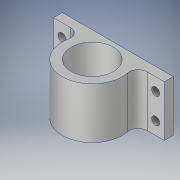
# Autodesk Inventor part: Motor Holder
Saved by Autodesk Inventor 2017 (Build 210142000, 142)
## iProperties
Created: 2017-01-31
Part Number: Motor Holder
Material: Aluminum 6061
Document SubType Name: Modeling
Designer: qupec
Density: 2.7 g/cm^3
Appearance: Aluminum - Flat
Author: qupec
Autodesk Inventor part; units mm, degrees
ref_plane "YZ Plane" through (0, 0, 0) normal (1, 0, 0) x (0, 1, 0)
ref_plane "XZ Plane" through (0, 0, 0) normal (0, 1, 0) x (-1, 0, 0)
sketch "Sketch1" plane through (0, 0, 0) normal (0, 1, 0) x (-1, 0, 0)
  circle A0 centre (0, 0) radius 7.5
  line L0 (0, -7.5) -> (0, -7.5) construction
  arc A1 (10.4644, -2.11) -> (-10.4644, -2.11) centre (0, 0) ccw
  line L1 (0, -9.0875) -> (-19.685, -9.0875)
  line L2 (-19.685, -9.0875) -> (-19.685, -5.9125)
  line L3 (-19.685, -5.9125) -> (-13.5768, -5.9125)
  arc A2 (-13.5768, -5.9125) -> (-10.4644, -2.11) centre (-13.5768, -2.7375) ccw
  line L4 (0, -9.0875) -> (0, 10.675) construction
  line L5 (0, -9.0875) -> (19.685, -9.0875)
  line L6 (19.685, -9.0875) -> (19.685, -5.9125)
  line L7 (19.685, -5.9125) -> (13.5768, -5.9125)
  arc A3 (10.4644, -2.11) -> (13.5768, -5.9125) centre (13.5768, -2.7375) ccw
  dimension "d0" = 15
  dimension "d33" = 3.175
  dimension "d34" = 1.5875
  dimension "d35" = 19.685
  dimension "d36" = 3.175
  dimension "d37" = 6.35
  constraints: 16 end point, 7 point on circle, 5 symmetric about line, 3 centre point, 2 coincident, 2 horizontal, 2 tangent, 1 perpendicular, 1 vertical, 1 vertical alignment, 3 other
  measures "d34" distance of L0.end L1.start
  measures "d35" distance of L1.start L1.end
  measures "d36" distance of L1.end L2.end
  measures "d37" diameter of A2
ref_plane "Work Plane1" through (-5.4205, 4.7625, -2.8174) normal (0, 0, 1) x (1, 0, 0)
extrude "Extrusion5" add sketch "Sketch1" along normal blind 15.5
sketch "Sketch7" plane through (0, 0, 0) normal (0, -1, 0) x (1, 0, 0)
  circle A0 centre (0, 0) radius 7.5 construction
  line L0 (-19.685, -9.0875) -> (19.685, -9.0875) projected
  line L1 (19.685, -9.0875) -> (19.685, -5.9125) projected
  line L2 (19.685, -5.9125) -> (13.5768, -5.9125) projected
  arc A1 (10.4644, -2.11) -> (13.5768, -5.9125) centre (13.5768, -2.7375) ccw projected
  arc A2 (10.4644, -2.11) -> (-10.4644, -2.11) centre (0, 0) ccw projected
  arc A3 (-13.5768, -5.9125) -> (-10.4644, -2.11) centre (-13.5768, -2.7375) ccw projected
  line L3 (-13.5768, -5.9125) -> (-19.685, -5.9125) projected
  line L4 (-19.685, -5.9125) -> (-19.685, -9.0875) projected
extrude "Extrusion6" add sketch "Sketch7" along normal blind 2.54
sketch "Sketch6" plane through (13.5768, 0, -5.9125) normal (0, 0, 1) x (1, 0, 0)
  line L0 (6.1082, 0) -> (0, 0) projected
  line L1 (6.1082, 0) -> (6.1082, 15.5) projected
  line L2 (0, 15.5) -> (0, -2.54) projected
  line L3 (-3.1124, 15.5) -> (0, 15.5) projected
  line L4 (-3.1124, 15.5) -> (-3.1124, -2.54) projected
  line L5 (0, 15.5) -> (6.1082, 15.5) projected
  line L6 (0, -2.54) -> (-3.1124, -2.54) projected
  line L7 (6.1082, -2.54) -> (0, -2.54) projected
  point P0 (-13.5768, 0)
  point P1 (3.0541, 1.97)
  point P2 (3.0541, 10.99)
  dimension "d42" = 3.0541
  dimension "d43" = 6.1082
  dimension "d44" = 3.0541
  dimension "d46" = 4.51
  dimension "d56" = 18.04
  dimension "d57" = 4.51
  measures "d42" distance from line of point (3.054, 1.97) L1
  measures "d43" distance between parallel lines of L2 L1
  measures "d44" distance from line of L1 point (3.054, 10.99)
  measures "d46" distance from line of point (3.054, 10.99) L5
  measures "d56" distance between parallel lines of L7 L5
  measures "d57" distance from line of L7 point (3.054, 1.97)
hole "Hole1" at (16.6309, 1.97, -5.9125) at (16.6309, 10.99, -5.9125) direction (0, 0, -1) diameter 2.8448 depth 25.4 tip angle 118
mirror "Mirror3" about plane through (0, 0, 0) normal (1, 0, 0) of "Hole1"
sketch "Sketch8" plane through (0, -2.54, 0) normal (0, -1, 0) x (1, 0, 0)
  circle A0 centre (-4.924, 0.868) radius 0.625
  circle A1 centre (1.71, 4.698) radius 0.625
  circle A2 centre (4.924, -0.868) radius 0.625
  circle A3 centre (-3.214, -3.83) radius 0.625
  circle A4 centre (0, 0) radius 3.1
  dimension "d58" = 1.25
  dimension "d59" = 1.25
  dimension "d60" = 1.25
  dimension "d61" = 1.25
  dimension "d62" = 4.924
  dimension "d63" = 0.868
  dimension "d64" = 3.83
  dimension "d65" = 3.214
  dimension "d66" = 1.71
  dimension "d67" = 4.698
  dimension "d68" = 0.868
  dimension "d69" = 4.924
  dimension "d72" = 6.2
  constraints: 5 centre point, 1 coincident
  measures "d58" diameter of A0
  measures "d59" diameter of A1
  measures "d60" diameter of A2
  measures "d61" diameter of A3
  measures "d62" horizontal distance of point (0, 0) A0.centre
  measures "d63" vertical distance of point (0, 0) A0.centre
  measures "d64" vertical distance of point (0, 0) A3.centre
  measures "d65" horizontal distance of point (0, 0) A3.centre
  measures "d66" horizontal distance of point (0, 0) A1.centre
  measures "d67" vertical distance of A1.centre point (0, 0)
  measures "d68" vertical distance of point (0, 0) A2.centre
  measures "d69" horizontal distance of point (0, 0) A2.centre
  measures "d72" diameter of A4
extrude "Extrusion7" cut sketch "Sketch8" against normal through all
equation "\"d42\" = 0.5 * d43"
equation "\"d44\" = 0.5 * d43"
equation "\"d46\" = d57"
equation "\"d57\" = 0.25 * d56"
equation "\"d59\" = d58"
equation "\"d60\" = d59"
equation "\"d61\" = d58"
equation "\"d41\" = 0.25 * d56"
body "Solid1"
